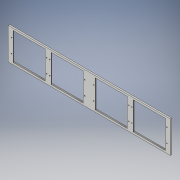
# Autodesk Inventor part: Ra-Manager_Painel_Traseiro
Saved by Autodesk Inventor 2019.4 (Build 234330000, 330)
## iProperties
Created: 2020-03-11
Part Number: Ra-Manager_Painel_Traseiro
Material: Aço, carbono
Document SubType Name: Modeling
Designer: caio.santos
Density: 7.85 g/cm^3
Appearance: Semipolido
Author: caio.santos
Autodesk Inventor part; units mm, degrees
ref_plane "YZ Plane" through (0, 0, 0) normal (1, 0, 0) x (0, 1, 0)
ref_plane "XZ Plane" through (0, 0, 0) normal (0, 1, 0) x (-1, 0, 0)
ref_plane "XY Plane" through (0, 0, 0) normal (0, 0, 1) x (1, 0, 0)
sketch "Esboço1" plane through (0, 0, 0) normal (0, 0, 1) x (1, 0, 0)
  line L0 (-215, -42) -> (215, -42)
  line L1 (215, -42) -> (215, 42)
  line L2 (215, 42) -> (-215, 42)
  line L3 (-215, 42) -> (-215, -42)
  point P0 (0, 0)
  dimension "d2" = 430
  dimension "d4" = 84
  dimension "d6" = 215
  dimension "d7" = 42
  constraints: 8 end point, 1 horizontal, 1 parallel, 1 perpendicular, 1 vertical
  measures "d2" distance of L0.start L0.end
  measures "d4" distance of L0.end L1.end
  measures "d6" distance from line of L3 point (0, 0)
  measures "d7" distance from line of point (0, 0) L2
extrude "Extrusão1" add sketch "Esboço1" against normal blind 4
sketch "Esboço3" plane through (0, 0, 0) normal (0, 0, 1) x (1, 0, 0)
  line L0 (-215, -42) -> (-215, 42) projected
  line L1 (215, -42) -> (-215, -42) projected
  line L2 (-215, 37) -> (215, 37) construction
  line L3 (-210, 42) -> (-210, -42) construction
  line L4 (210, 42) -> (210, -42) construction
  line L5 (-215, -37) -> (215, -37) construction
  line L6 (-8, 37) -> (-8, -37) construction
  line L7 (8, 37) -> (8, -37) construction
  line L8 (210, 37) -> (210, -37)
  line L9 (-202, 37) -> (-202, -37)
  line L10 (-16, 37) -> (-16, -37)
  line L11 (-117, 37) -> (-117, -37)
  line L12 (-101, 37) -> (-101, -37)
  line L13 (16, 37) -> (16, -37)
  line L14 (202, 37) -> (202, -37)
  line L15 (101, 37) -> (101, -37)
  line L16 (117, 37) -> (117, -37)
  line L17 (-202, -37) -> (-117, -37)
  line L18 (-202, 37) -> (-117, 37)
  line L19 (-101, 37) -> (-16, 37)
  line L20 (-16, -37) -> (-101, -37)
  line L21 (202, 37) -> (117, 37)
  line L22 (101, 37) -> (16, 37)
  line L23 (-215, 42) -> (215, 42) projected
  line L24 (16, -37) -> (101, -37)
  line L25 (117, -37) -> (202, -37)
  point P0 (0, 0)
  dimension "d79" = 79
  dimension "d80" = 5
  dimension "d81" = 79
  dimension "d82" = 5
  dimension "d83" = 79
  dimension "d84" = 5
  dimension "d85" = 79
  dimension "d86" = 5
  dimension "d87" = 199
  dimension "d88" = 114
  dimension "d89" = 98
  dimension "d90" = 13
  dimension "d91" = 79
  dimension "d92" = 5
  dimension "d93" = 425
  dimension "d94" = 417
  dimension "d95" = 332
  dimension "d96" = 316
  dimension "d97" = 231
  dimension "d98" = 223
  dimension "d99" = 207
  dimension "d100" = 5
  dimension "d101" = 430
  dimension "d102" = 430
  dimension "d103" = 84
  dimension "d104" = 84
  constraints: 46 end point, 12 point on line, 10 perpendicular, 7 collinear, 3 parallel, 2 horizontal
  measures "d79" distance between parallel lines of L1 L22
  measures "d80" distance between parallel lines of L1 L24
  measures "d81" distance between parallel lines of L1 L2
  measures "d82" distance between parallel lines of L1 L5
  measures "d83" distance between parallel lines of L1 L19
  measures "d84" distance between parallel lines of L1 L20
  measures "d85" distance between parallel lines of L1 L18
  measures "d86" distance between parallel lines of L1 L17
  measures "d87" distance between parallel lines of L0 L10
  measures "d88" distance between parallel lines of L0 L12
  measures "d89" distance between parallel lines of L0 L11
  measures "d90" distance between parallel lines of L0 L9
  measures "d91" distance between parallel lines of L21 L1
  measures "d92" distance between parallel lines of L25 L1
  measures "d93" distance between parallel lines of L8 L0
  measures "d94" distance between parallel lines of L14 L0
  measures "d95" distance between parallel lines of L16 L0
  measures "d96" distance between parallel lines of L15 L0
  measures "d97" distance between parallel lines of L13 L0
  measures "d98" distance between parallel lines of L7 L0
  measures "d99" distance between parallel lines of L6 L0
  measures "d100" distance between parallel lines of L3 L0
  measures "d101" distance from line of L2.end L0
  measures "d102" distance from line of L5.end L0
  measures "d103" distance from line of L4.start L1
  measures "d104" distance from line of L3.start L1
extrude "Extrusão2" cut sketch "Esboço3" against normal blind 10
sketch "Esboço5" plane through (0, 0, -4) normal (0, 0, -1) x (-1, 0, 0)
  line L0 (-215, 37) -> (215, 37) construction
  line L1 (-210, 42) -> (-210, -42) construction
  line L2 (210, 42) -> (210, -42) construction
  line L3 (-215, -37) -> (215, -37) construction
  line L4 (-8, 37) -> (-8, -37) construction
  line L5 (8, 37) -> (8, -37) construction
  line L6 (-117, -37) -> (-202, -37)
  line L7 (-202, -37) -> (-210, -37)
  line L8 (-210, 37) -> (-210, -37)
  line L9 (-210, 37) -> (-202, 37)
  line L10 (-202, 37) -> (-117, 37)
  line L11 (-202, 37) -> (-202, -37)
  line L12 (-101, 37) -> (-16, 37)
  line L13 (-117, 37) -> (-101, 37)
  line L14 (-101, -37) -> (-101, 37)
  line L15 (-101, 37) -> (-101, -37)
  line L16 (-101, -37) -> (-117, -37)
  line L17 (-117, 37) -> (-117, -37)
  line L18 (-16, 37) -> (-8, 37)
  line L19 (-8, 37) -> (-8, -37)
  line L20 (-8, -37) -> (-16, -37)
  line L21 (-16, 37) -> (-16, -37)
  line L22 (-16, -37) -> (-16, 37)
  line L23 (16, 37) -> (101, 37)
  line L24 (8, 37) -> (16, 37)
  line L25 (16, -37) -> (16, 37)
  line L26 (16, 37) -> (16, -37)
  line L27 (16, -37) -> (8, -37)
  line L28 (8, 37) -> (8, -37)
  line L29 (101, 37) -> (101, -37)
  line L30 (101, 37) -> (117, 37)
  line L31 (117, -37) -> (117, 37)
  line L32 (117, 37) -> (117, -37)
  line L33 (117, -37) -> (101, -37)
  line L34 (101, -37) -> (101, 37)
  line L35 (117, 37) -> (202, 37)
  line L36 (202, 37) -> (210, 37)
  line L37 (210, -37) -> (210, 37)
  line L38 (202, -37) -> (117, -37)
  line L39 (202, 37) -> (202, -37)
  line L40 (202, -37) -> (210, -37)
  point P0 (0, 0)
  point P1 (0, 0)
  point P2 (0, 0)
  dimension "d188" = 109
  dimension "d189" = 109
  dimension "d190" = 125
  dimension "d191" = 327
  dimension "d192" = 98
  dimension "d193" = 98
  dimension "d194" = 79
  dimension "d195" = 5
  dimension "d196" = 37
  dimension "d197" = 117
  dimension "d198" = 79
  dimension "d199" = 5
  dimension "d200" = 332
  dimension "d201" = 332
  dimension "d202" = 90
  dimension "d203" = 90
  dimension "d204" = 90
  dimension "d205" = 90
  dimension "d206" = 8
  dimension "d207" = 93
  dimension "d208" = 194
  dimension "d209" = 226
  dimension "d210" = 311
  dimension "d211" = 327
  dimension "d212" = 412
  dimension "d213" = 74
  dimension "d214" = 210
  dimension "d215" = 37
  dimension "d216" = 74
  dimension "d217" = 210
  dimension "d218" = 37
  constraints: 78 end point, 6 horizontal, 5 collinear, 5 perpendicular, 5 vertical, 4 point on line, 3 parallel, 17 other
  measures "d188" distance between parallel lines of L29 L37
  measures "d189" distance between parallel lines of L31 L28
  measures "d190" distance between parallel lines of L31 L19
  measures "d191" distance between parallel lines of L31 L1
  measures "d192" distance from line of point (215, 37) L31
  measures "d193" distance from line of point (215, -37) L31
  measures "d194" distance from line of L2.start L38
  measures "d195" distance from line of L2.end L38
  measures "d196" distance from line of point (0, 0) L38
  measures "d197" distance from line of point (0, 0) L31
  measures "d198" distance from line of L1.start L38
  measures "d199" distance from line of L1.end L38
  measures "d200" distance from line of point (-215, 37) L31
  measures "d201" distance from line of point (-215, -37) L31
  measures "d202" angle of L36 L37
  measures "d203" angle of L37 L38
  measures "d204" angle of L2 L18
  measures "d205" angle of L6 L2
  measures "d206" distance between parallel lines of L37 L39
  measures "d207" distance between parallel lines of L37 L31
  measures "d208" distance between parallel lines of L25 L37
  measures "d209" distance between parallel lines of L21 L37
  measures "d210" distance between parallel lines of L15 L37
  measures "d211" distance between parallel lines of L17 L37
  measures "d212" distance between parallel lines of L11 L37
  measures "d214" distance from line of point (0, 0) L37
  measures "d215" distance from line of point (0, 0) L36
  measures "d216" distance from line of L29.end L36
  measures "d217" distance from line of point (0, 0) L37
  measures "d218" distance from line of point (0, 0) L36
extrude "Extrusão4" cut sketch "Esboço5" against normal blind 2
sketch "Esboço6" plane through (0, 0, -2) normal (0, 0, -1) x (-1, 0, 0)
  line L0 (-210, 37) -> (-202, 37) projected
  line L1 (-210, 37) -> (-8, 37) projected
  line L2 (-210, -37) -> (-210, 37) projected
  line L3 (-210, 18.5) -> (210, 18.5) construction
  line L4 (210, 37) -> (210, -37) projected
  line L5 (-210, -18.5) -> (210, -18.5) construction
  line L6 (-117, 37) -> (-101, 37) projected
  line L7 (-206, 37) -> (-206, -37) construction
  line L8 (-113, 37) -> (-113, -37) construction
  line L9 (-105, 37) -> (-105, -37) construction
  line L10 (8, 37) -> (16, 37) projected
  line L11 (12, 37) -> (12, -37) construction
  line L12 (-16, 37) -> (-8, 37) projected
  line L13 (-12, 37) -> (-12, -37) construction
  line L14 (-8, -37) -> (-16, -37) projected
  line L15 (101, 37) -> (117, 37) projected
  line L16 (105, 37) -> (105, -37) construction
  line L17 (113, 37) -> (113, -37) construction
  line L18 (202, 37) -> (210, 37) projected
  line L19 (206, 37) -> (206, -37) construction
  line L20 (210, -37) -> (8, -37) projected
  point P0 (0, 0)
  point P1 (-206, 18.5)
  point P2 (-206, -18.5)
  point P3 (-113, -18.5)
  point P4 (-105, -18.5)
  point P5 (-113, 18.5)
  point P6 (-105, 18.5)
  point P7 (-12, 18.5)
  point P8 (-12, -18.5)
  point P9 (12, -18.5)
  point P10 (12, 18.5)
  point P11 (105, 18.5)
  point P12 (113, 18.5)
  point P13 (113, -18.5)
  point P14 (105, -18.5)
  point P15 (206, 18.5)
  point P16 (206, -18.5)
  dimension "d230" = 18.5
  dimension "d231" = 55.5
  dimension "d232" = 97
  dimension "d233" = 105
  dimension "d234" = 315
  dimension "d235" = 323
  dimension "d236" = 416
  dimension "d237" = 0
  dimension "d238" = 0
  dimension "d239" = 0
  dimension "d240" = 0
  dimension "d241" = 74
  dimension "d242" = 0
  constraints: 26 point on line, 16 end point, 6 vertical, 4 midpoint, 1 parallel, 1 perpendicular, 22 other
  measures "d232" distance between parallel lines of L17 L4
  measures "d233" distance between parallel lines of L16 L4
  measures "d234" distance between parallel lines of L9 L4
  measures "d235" distance between parallel lines of L8 L4
  measures "d236" distance between parallel lines of L7 L4
  measures "d237" distance from line of L17.end L14
  measures "d238" distance from line of L16.end L20
  measures "d239" distance from line of L11.end L20
  measures "d240" distance from line of L9.end L20
  measures "d241" distance from line of L8.end L1
  measures "d242" distance from line of L7.end L14
hole "Furo1" at (206, 18.5, -2) at (206, -18.5, -2) at (113, -18.5, -2) at (105, -18.5, -2) at (113, 18.5, -2) at (105, 18.5, -2) at (12, 18.5, -2) at (12, -18.5, -2) at (-12, -18.5, -2) at (-12, 18.5, -2) at (-105, 18.5, -2) at (-113, 18.5, -2) at (-113, -18.5, -2) at (-105, -18.5, -2) at (-206, 18.5, -2) at (-206, -18.5, -2) direction (0, 0, 1) diameter 2.459 end through all thread size "M3x0.5" class "6H" standard "ANSI Metric M Profile"
equation "\"d2\" = 2 * d6"
equation "\"d4\" = 2 * d7"
